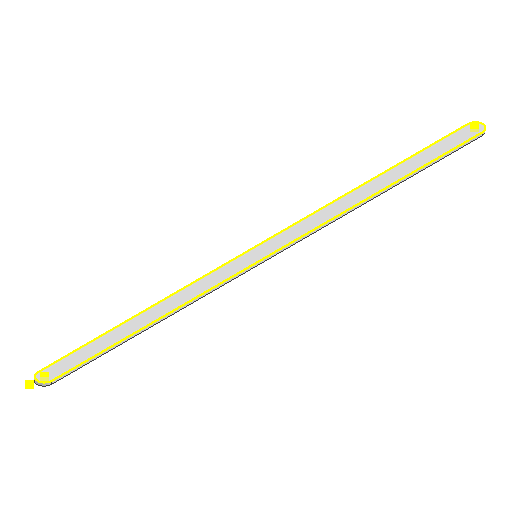
# Autodesk Inventor part: Wing_arm_3_reinforcement
Saved by Autodesk Inventor 2022 (Build 260153000, 153)
## iProperties
Created: 2022-07-07
Part Number: Wing_arm_3_reinforcement
Material: Generic
Document SubType Name: Modeling
Designer: dell
Density: 1 g/cm^3
Appearance: Default
Author: dell
Autodesk Inventor part; units mm, degrees
ref_plane "YZ Plane" through (0, 0, 0) normal (1, 0, 0) x (0, 1, 0)
ref_plane "XZ Plane" through (0, 0, 0) normal (0, 1, 0) x (-1, 0, 0)
ref_plane "XY Plane" through (0, 0, 0) normal (0, 0, 1) x (1, 0, 0)
sketch "Sketch1" plane through (0, 0, 0) normal (0, 1, 0) x (-1, 0, 0)
  line L0 (0, 0) -> (0, -263.803) construction
  line L1 (-4, 0) -> (-4, -263.803)
  line L2 (4, -263.803) -> (4, 0)
  arc A0 (4, 0) -> (-4, 0) centre (0, 0) ccw
  arc A1 (-4, -263.803) -> (4, -263.803) centre (0, -263.803) ccw
  circle A2 centre (0, 0) radius 1.5
  circle A3 centre (0, -263.803) radius 1.5
  point P0 (0, -131.9015)
  dimension "d0" = 263.803
  dimension "d1" = 8
  dimension "d2" = 3
  dimension "d3" = 3
  constraints: 8 end point, 4 centre point, 4 point on circle, 4 tangent, 2 coincident, 1 midpoint, 1 parallel, 1 vertical
  measures "d0" distance of L0.start L0.end
  measures "d1" diameter of A1
  measures "d2" diameter of A2
  measures "d3" diameter of A3
extrude "Extrusion1" add sketch "Sketch1" along normal blind 4.5
sketch "Sketch2" plane through (0, 4.5, 0) normal (0, 1, 0) x (1, 0, 0)
  line L0 (0, 8) -> (0, 247.803) construction
  line L1 (4, 8) -> (4, 247.803)
  line L2 (-4, 247.803) -> (-4, 8)
  arc A0 (-4, 8) -> (4, 8) centre (0, 8) ccw
  arc A1 (4, 247.803) -> (-4, 247.803) centre (0, 247.803) ccw
  arc A2 (4, 263.803) -> (-4, 263.803) centre (0, 263.803) ccw projected
  line L3 (-4, 263.803) -> (-4, 0) projected
  arc A3 (-4, 0) -> (4, 0) centre (0, 0) ccw projected
  line L4 (4, 0) -> (4, 263.803) projected
  circle A4 centre (0, 263.803) radius 1.5 projected
  circle A5 centre (0, 0) radius 1.5 projected
  point P0 (0, 127.9015)
  point P1 (-4, 8)
  dimension "d6" = 8
  dimension "d7" = 16
  dimension "d8" = 8
  constraints: 8 end point, 4 point on circle, 4 tangent, 2 centre point, 1 midpoint, 1 parallel, 1 point on line, 1 vertical
  measures "d6" diameter of A1
  measures "d7" distance of A2.centre L0.end
  measures "d8" distance of L0.start point (0, 0)
extrude "Extrusion2" add sketch "Sketch2" along normal blind 2 contours A0 L2 A1 L1
extrude "Extrusion3" cut sketch "Sketch2" against normal blind 100
sketch "Sketch3" plane through (0, 6.5, 0) normal (0, 1, 0) x (1, 0, 0)
  line L0 (4, 8) -> (4, 247.803) projected
  line L1 (-4, 247.803) -> (-4, 8) projected
  arc A0 (-4, 8) -> (4, 8) centre (0, 8) ccw projected
  line L2 (4, 8) -> (4, 247.803) projected
  arc A1 (4, 247.803) -> (-4, 247.803) centre (0, 247.803) ccw projected
  point P0 (0, 0)
body "Solid1"
